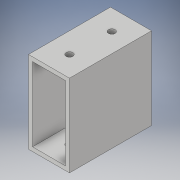
# Autodesk Inventor part: Pulley_holder
Saved by Autodesk Inventor 2018 (Build 220112000, 112)
## iProperties
Created: 2018-08-30
Part Number: Pulley_holder
Material: Generic
Document SubType Name: Modeling
Designer: baoan
Density: 1 g/cm^3
Appearance: Default
Author: baoan
Autodesk Inventor part; units mm, degrees
ref_plane "YZ Plane" through (0, 0, 0) normal (1, 0, 0) x (0, 1, 0)
ref_plane "XZ Plane" through (0, 0, 0) normal (0, 1, 0) x (-1, 0, 0)
ref_plane "XY Plane" through (0, 0, 0) normal (0, 0, 1) x (1, 0, 0)
sketch "Sketch1" plane through (0, 0, 0) normal (0, 0, 1) x (1, 0, 0)
  line L0 (-12.7, -25.4) -> (12.7, -25.4)
  line L1 (12.7, -25.4) -> (12.7, 25.4)
  line L2 (12.7, 25.4) -> (-12.7, 25.4)
  line L3 (-12.7, 25.4) -> (-12.7, -25.4)
  line L4 (-12.7, -25.4) -> (12.7, 25.4) construction
  line L5 (12.7, -25.4) -> (-12.7, 25.4) construction
  line L6 (-10.16, -22.86) -> (10.16, -22.86)
  line L7 (10.16, -22.86) -> (10.16, 22.86)
  line L8 (10.16, 22.86) -> (-10.16, 22.86)
  line L9 (-10.16, 22.86) -> (-10.16, -22.86)
  line L10 (-10.16, -22.86) -> (10.16, 22.86) construction
  line L11 (10.16, -22.86) -> (-10.16, 22.86) construction
  point P0 (0, 0)
  dimension "d0" = 25.4
  dimension "d1" = 50.8
  dimension "d2" = 20.32
  dimension "d3" = 45.72
  constraints: 24 end point, 4 midpoint, 4 parallel, 2 horizontal, 2 perpendicular
  measures "d0" distance of L2.end L1.end
  measures "d1" distance of L1.end L0.end
  measures "d2" distance of L8.end L7.end
  measures "d3" distance of L7.end L6.end
extrude "Extrusion1" add sketch "Sketch1" along normal mid plane 50.8
sketch "Sketch2" plane through (-12.7, 25.4, 25.4) normal (0, 1, 0) x (1, 0, 0)
  line L0 (25.4, 0) -> (0, 0) projected
  line L1 (25.4, 50.8) -> (25.4, 0) projected
  point P0 (12.7, 25.4)
  point P1 (12.7, 12.7)
  point P2 (13.5104, 38.1)
  dimension "d6" = 25.4
  dimension "d7" = 12.7
  dimension "d8" = 12.7
  measures "d6" vertical distance of point (13.51, 38.1) point (12.7, 12.7)
  measures "d7" distance from line of L0 point (12.7, 12.7)
  measures "d8" distance from line of L1 point (12.7, 12.7)
hole "Hole1" at (0, 25.4, 12.7) at (0.8104, 25.4, -12.7) direction (0, -1, 0) diameter 4.1402 end through all
body "Solid1"
